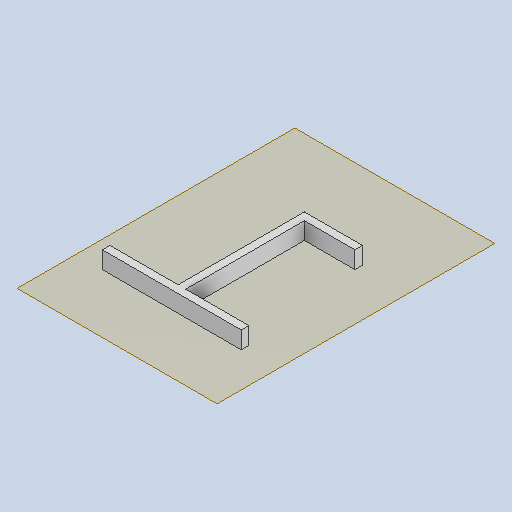
# Autodesk Inventor part: battery_holder
Saved by Autodesk Inventor 2022 (Build 260153000, 153)
## iProperties
Created: 2021-12-09
Part Number: battery_holder
Material: Generic
Document SubType Name: Modeling
Designer: simen
Density: 1 g/cm^3
Appearance: Default
Author: simen
## iProperties of the stored document battery_holder_3DPrint.ipt
Created: 2021-12-09
Part Number: battery_holder_3DPrint
Material: Generic
Document SubType Name: Modeling
Designer: simen
Density: 1 g/cm^3
Appearance: Default
Author: simen
Autodesk Inventor part; units mm, degrees
ref_plane "YZ Plane" through (0, 0, 0) normal (1, 0, 0) x (0, 1, 0)
ref_plane "XZ Plane" through (0, 0, 0) normal (0, 1, 0) x (-1, 0, 0)
ref_plane "XY Plane" through (0, 0, 0) normal (0, 0, 1) x (1, 0, 0)
ref_plane "Work Plane1" through (182.8917, 65.9403, 21.7484) normal (0, 1, 0) x (0, 0, -1)
sketch "Sketch1" plane through (182.8917, 65.9403, 21.7484) normal (0, 1, 0) x (0, 0, -1)
  line L0 (-78.6913, -1.8576) -> (-78.6913, -56.8576)
  line L1 (-78.6913, -56.8576) -> (-75.6913, -56.8576)
  line L2 (-75.6913, -56.8576) -> (-75.6913, -31.8576)
  line L3 (-75.6913, -31.8576) -> (-28.6913, -31.8576)
  line L4 (-28.6913, -31.8576) -> (-28.6913, -28.8576)
  line L5 (-28.6913, -31.8576) -> (-28.6913, -51.8576)
  line L6 (-28.6913, -51.8576) -> (-25.6913, -51.8576)
  line L7 (-25.6913, -51.8576) -> (-25.6913, -28.8576)
  line L8 (-25.6913, -28.8576) -> (-75.6913, -28.8576)
  line L9 (-75.6913, -28.8576) -> (-75.6913, -1.8576)
  line L10 (-75.6913, -1.8576) -> (-78.6913, -1.8576)
  point P0 (21.7484, 182.8917)
  dimension "d0" = 55
  dimension "d1" = 3
  dimension "d2" = 25
  dimension "d3" = 47
  dimension "d4" = 3
  dimension "d5" = 3
  dimension "d6" = 23
  constraints: 22 end point, 9 perpendicular, 2 vertical, 1 collinear
  measures "d0" distance of L0.start L0.end
  measures "d1" distance of L0.end L1.end
  measures "d2" distance of L1.end L2.end
  measures "d3" distance of L2.end L3.end
  measures "d4" distance of L3.end L4.end
  measures "d5" distance of L5.end L6.end
  measures "d6" distance of L6.end L7.end
extrude "Extrusion1" add sketch "Sketch1" along normal blind 6.8
body "Solid1"
